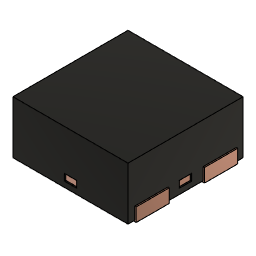
DPW0005A v3 (Autodesk Fusion 360 design; units mm, degrees)
Autodesk Fusion 360 part; units mm, degrees
sketch "Sketch1" plane through (0, 0, 0) normal (0, 0, 1) x (1, 0, 0)
  line L0 (0, 0) -> (0.85, 0)
  line L1 (0.85, 0) -> (0.85, 0.85)
  line L2 (0.85, 0.85) -> (0, 0.85)
  line L3 (0, 0.85) -> (0, 0)
  dimension "d1" = 0.85
  dimension "d2" = 0.85
  constraint horizontal L0
  constraint vertical L1
  constraint horizontal L2
  constraint vertical L3
  constraint coincident L0.start L3.end
  measures "d1" distance of L0.start L0.end
  measures "d2" distance of L0.start L2.end
extrude "Extrude1" add sketch "Sketch1" along normal blind 0.4
sketch "Sketch2" plane through (0, 0, 0) normal (0, 0, -1) x (1, 0, 0)
  line L0 (0, 0) -> (0, -0.85)
  line L1 (0, -0.85) -> (0.85, -0.85)
  line L2 (0.85, -0.85) -> (0.85, 0)
  line L3 (0.85, 0) -> (0, 0)
  line L4 (0.425, -0.85) -> (0.85, -0.85)
  line L5 (0.425, -0.85) -> (0.425, 0)
  line L6 (0.425, -0.425) -> (0.85, -0.425)
  line L7 (0.425, -0.425) -> (0, -0.425)
  line L8 (0.425, -0.425) -> (0.425, -0.241)
  line L9 (0.425, -0.425) -> (0.425, -0.609)
  line L10 (0.425, -0.425) -> (0.609, -0.425)
  line L11 (0.425, -0.425) -> (0.241, -0.425)
  line L12 (0.241, -0.425) -> (0.425, -0.241)
  line L13 (0.425, -0.241) -> (0.609, -0.425)
  line L14 (0.609, -0.425) -> (0.425, -0.609)
  line L15 (0.425, -0.609) -> (0.241, -0.425)
  line L16 (0, -0.425) -> (0, -0.555)
  line L17 (0, -0.425) -> (0, -0.295)
  line L18 (0.85, -0.425) -> (0.85, -0.295)
  line L19 (0.85, -0.425) -> (0.85, -0.555)
  line L20 (0.425, -0.85) -> (0.425, -0.75)
  line L21 (0.85, -0.425) -> (0.75, -0.425)
  line L22 (0.425, -0.75) -> (0.75, -0.425)
  line L23 (0.425, 0) -> (0.425, -0.1)
  line L24 (0.425, -0.1) -> (0.75, -0.425)
  line L25 (0, -0.425) -> (0.1, -0.425)
  line L26 (0.1, -0.425) -> (0.425, -0.1)
  line L27 (0.1, -0.425) -> (0.425, -0.75)
  line L28 (0, -0.555) -> (0.85, -0.555)
  line L29 (0.85, -0.295) -> (0, -0.295)
  line L30 (0, -0.85) -> (0, -0.8)
  line L31 (0, -0.8) -> (0.85, -0.8)
  line L32 (0.85, 0) -> (0.85, -0.05)
  line L33 (0, -0.05) -> (0.85, -0.05)
  line L34 (0.85, -0.05) -> (0, -0.05)
  line L35 (0.85, -0.8) -> (0.562, -0.8)
  line L36 (0, -0.8) -> (0.288, -0.8)
  line L37 (0, -0.05) -> (0.288, -0.05)
  line L38 (0.85, -0.05) -> (0.562, -0.05)
  line L39 (0.562, -0.8) -> (0.85, -0.512)
  line L40 (0.562, -0.8) -> (0.9693, -0.8) construction
  line L41 (0.288, -0.8) -> (0, -0.512)
  line L42 (0.562, -0.05) -> (0.85, -0.338)
  line L43 (0.288, -0.05) -> (0, -0.338)
  line L44 (0, -0.8) -> (0.239, -0.8)
  line L45 (0.239, -0.8) -> (0.239, -0.751)
  dimension "d7" = 0.184
  dimension "d8" = 0.184
  dimension "d9" = 0.184
  dimension "d10" = 0.184
  dimension "d11" = 0.13
  dimension "d12" = 0.13
  dimension "d13" = 0.13
  dimension "d14" = 0.13
  dimension "d15" = 0.288
  dimension "d16" = 0.288
  dimension "d17" = 0.288
  dimension "d18" = 0.288
  dimension "d19" = 45
  dimension "d20" = 90
  dimension "d21" = 90
  dimension "d22" = 0.239
  constraint midpoint L1 L4.start
  constraint coincident L1.end L2.start
  constraint perpendicular L4 L5
  constraint midpoint L5 L6.start
  constraint midpoint L2 L6.end
  constraint midpoint L0 L7.end
  constraint perpendicular L0 L7
  constraint perpendicular L7 L8
  constraint coincident L5 L9.end
  constraint perpendicular L5 L10
  constraint perpendicular L9 L11
  constraint perpendicular L7 L16
  constraint perpendicular L7 L17
  constraint perpendicular L6 L18
  constraint perpendicular L6 L19
  constraint coincident L5 L20.end
  constraint coincident L6 L21.end
  constraint coincident L5 L23.end
  constraint coincident L7 L25.end
  constraint coincident L0.end L1.start
  constraint coincident L0 L30.end
  constraint coincident L2 L31.end
  constraint perpendicular L2 L31
  constraint coincident L2.end L3.start
  constraint coincident L2 L32.end
  constraint perpendicular L3 L32
  constraint coincident L0 L33.start
  constraint perpendicular L2 L33
  constraint perpendicular L2 L35
  constraint perpendicular L30 L36
  constraint perpendicular L0 L37
  constraint perpendicular L32 L38
  constraint horizontal L40
  constraint coincident L19 L39.end
  constraint coincident L16 L41.end
  constraint coincident L18 L42.end
  constraint coincident L36 L44.end
  constraint coincident L41 L45.end
  constraint perpendicular L44 L45
  measures "d7" distance of L6.start L8.end
  measures "d8" distance of L6.start L9.end
  measures "d9" distance of L6.start L10.end
  measures "d10" distance of L6.start L11.end
  measures "d11" distance of L7.end L16.end
  measures "d12" distance of L7.end L17.end
  measures "d13" distance of L6.end L18.end
  measures "d14" distance of L6.end L19.end
  measures "d15" distance of L31.end L35.end
  measures "d16" distance of L30.end L36.end
  measures "d17" distance of L33.start L37.end
  measures "d18" distance of L32.end L38.end
  measures "d19" angle of L39 L40
  measures "d20" angle of L39 L41
  measures "d21" angle of L42 L43
  measures "d22" distance of L30.end L44.end
extrude "Extrude2" cut sketch "Sketch2" against normal blind 0.01 contours L0 L3 L5 L23 L33 L34 L37 | L2 L3 L5 L23 L32 L33 L34 L38 | L0 L17 L29 L43 | L5 L23 L26 L29 L33 L34 L43 | L5 L23 L24 L29 L33 L34 L42 | L0 L7 L17 L25 L26 L29 L43 | L5 L13 L24 L29 | L5 L12 L26 L29 | L0 L7 L16 L25 L27 L28 L41 | L7 L12 L26 L29 | L2 L18 L29 L42 | L2 L6 L18 L21 L24 L29 L42 | L6 L13 L24 L29 | L0 L16 L28 L41 | L7 L15 L27 L28 | L6 L14 L22 L28 | L2 L6 L19 L21 L22 L28 L39 | L5 L20 L27 L28 L31 L41 | L5 L15 L27 L28 | L5 L20 L22 L28 L31 L39 | L5 L14 L22 L28 | L0 L1 L5 L20 L30 L31 L36 L44 | L31 L36 L41 L45 | L2 L19 L28 L39 | L1 L2 L4 L5 L20 L31 L35
sketch "Sketch3" plane through (0, 0, 0) normal (-1, 0, 0) x (0, -1, 0)
  line L0 (-0.05, 0.01) -> (0, 0.01)
  line L1 (0, 0.01) -> (0, 0.4)
  line L2 (0, 0.4) -> (-0.85, 0.4)
  line L3 (-0.85, 0.4) -> (-0.85, 0.01)
  line L4 (-0.85, 0.01) -> (-0.8, 0.01)
  line L5 (-0.8, 0.01) -> (-0.8, 0)
  line L6 (-0.8, 0) -> (-0.555, 0)
  line L7 (-0.555, 0) -> (-0.555, 0.01)
  line L8 (-0.555, 0.01) -> (-0.295, 0.01)
  line L9 (-0.295, 0.01) -> (-0.295, 0)
  line L10 (-0.295, 0) -> (-0.05, 0)
  line L11 (-0.05, 0) -> (-0.05, 0.01)
  line L12 (-0.8, 0.01) -> (-0.8, 0.1)
  line L13 (-0.555, 0.01) -> (-0.555, 0.1)
  line L14 (-0.555, 0.1) -> (-0.8, 0.1)
  line L15 (-0.295, 0.01) -> (-0.295, 0.1)
  line L16 (-0.295, 0.1) -> (-0.05, 0.1)
  line L17 (-0.05, 0.1) -> (-0.05, 0.01)
  line L18 (-0.555, 0.1) -> (-0.47, 0.1)
  line L19 (-0.295, 0.1) -> (-0.38, 0.1)
  line L20 (-0.38, 0.1) -> (-0.47, 0.1)
  line L21 (-0.47, 0.1) -> (-0.47, 0.05)
  line L22 (-0.47, 0.05) -> (-0.38, 0.05)
  line L23 (-0.38, 0.05) -> (-0.38, 0.1)
  line L24 (-0.05, 0.1) -> (0, 0.1)
  line L25 (-0.8, 0.1) -> (-0.85, 0.1)
  dimension "d25" = 0.09
  constraint coincident L4.end L5.start
  constraint perpendicular L4 L12
  constraint coincident L7.end L8.start
  constraint perpendicular L8 L13
  constraint perpendicular L13 L14
  constraint coincident L8.end L9.start
  constraint perpendicular L8 L15
  constraint perpendicular L15 L16
  constraint coincident L0.start L11.end
  constraint perpendicular L15 L18
  constraint perpendicular L15 L19
  constraint perpendicular L15 L20
  constraint perpendicular L8 L21
  constraint perpendicular L21 L22
  constraint perpendicular L8 L23
  constraint coincident L1 L24.end
  constraint perpendicular L1 L24
  constraint coincident L3 L25.end
  constraint perpendicular L3 L25
  measures "d25" distance of L4.end L12.end
sketch "Sketch4" plane through (0, 0.85, 0) normal (0, 1, 0) x (-1, 0, 0)
  line L0 (-0.85, 0.01) -> (0, 0.01)
  line L1 (0, 0.01) -> (0, 0.4)
  line L2 (0, 0.4) -> (-0.85, 0.4)
  line L3 (-0.85, 0.4) -> (-0.85, 0.01)
  line L4 (0, 0.1) -> (-0.85, 0.1)
  line L5 (-0.425, 0.1) -> (-0.38, 0.1)
  line L6 (-0.425, 0.1) -> (-0.47, 0.1)
  line L7 (-0.47, 0.1) -> (-0.47, 0.05)
  line L8 (-0.47, 0.05) -> (-0.38, 0.05)
  line L9 (-0.38, 0.05) -> (-0.38, 0.1)
  constraint coincident L1 L4.start
  constraint coincident L3 L4.end
  constraint perpendicular L3 L4
  constraint midpoint L4 L5.start
  constraint coincident L4 L5.end
  constraint perpendicular L3 L5
  constraint coincident L4 L6.end
  constraint perpendicular L3 L6
  constraint perpendicular L5 L7
  constraint perpendicular L7 L8
  constraint perpendicular L8 L9
sketch "Sketch5" plane through (0, 0, 0) normal (0, -1, 0) x (1, 0, 0)
  line L0 (0, 0.01) -> (0.85, 0.01)
  line L1 (0.85, 0.01) -> (0.85, 0.4)
  line L2 (0.85, 0.4) -> (0, 0.4)
  line L3 (0, 0.4) -> (0, 0.01)
  line L4 (0, 0.1) -> (0.85, 0.1)
  line L5 (0.425, 0.1) -> (0.47, 0.1)
  line L6 (0.47, 0.1) -> (0.47, 0.05)
  line L7 (0.47, 0.05) -> (0.38, 0.05)
  line L8 (0.38, 0.05) -> (0.38, 0.1)
  constraint coincident L3 L4.start
  constraint coincident L1 L4.end
  constraint perpendicular L1 L4
  constraint midpoint L4 L5.start
  constraint coincident L4 L5.end
  constraint parallel L4 L5
  constraint perpendicular L4 L6
  constraint perpendicular L6 L7
  constraint coincident L4 L8.end
  constraint perpendicular L4 L8
sketch "Sketch6" plane through (0.85, 0, 0) normal (1, 0, 0) x (0, 1, 0)
  line L0 (0, 0.01) -> (0.05, 0.01)
  line L1 (0.05, 0.01) -> (0.05, 0)
  line L2 (0.05, 0) -> (0.295, 0)
  line L3 (0.295, 0) -> (0.295, 0.01)
  line L4 (0.295, 0.01) -> (0.555, 0.01)
  line L5 (0.555, 0.01) -> (0.555, 0)
  line L6 (0.555, 0) -> (0.8, 0)
  line L7 (0.8, 0) -> (0.8, 0.01)
  line L8 (0.8, 0.01) -> (0.85, 0.01)
  line L9 (0.85, 0.01) -> (0.85, 0.4)
  line L10 (0.85, 0.4) -> (0, 0.4)
  line L11 (0, 0.4) -> (0, 0.01)
  line L12 (0, 0.1) -> (0.85, 0.1)
  line L13 (0.425, 0.1) -> (0.47, 0.1)
  line L14 (0.47, 0.1) -> (0.47, 0.05)
  line L15 (0.47, 0.05) -> (0.38, 0.05)
  line L16 (0.38, 0.05) -> (0.38, 0.1)
  line L17 (0.555, 0.01) -> (0.555, 0.1)
  line L18 (0.8, 0.01) -> (0.8, 0.1)
  line L19 (0.295, 0.01) -> (0.295, 0.1)
  line L20 (0.05, 0.01) -> (0.05, 0.1)
  constraint coincident L11 L12.start
  constraint coincident L9 L12.end
  constraint perpendicular L9 L12
  constraint midpoint L12 L13.start
  constraint coincident L12 L13.end
  constraint perpendicular L9 L13
  constraint perpendicular L13 L14
  constraint perpendicular L9 L15
  constraint coincident L12 L16.end
  constraint perpendicular L12 L16
  constraint coincident L4.end L5.start
  constraint perpendicular L4 L17
  constraint coincident L7.end L8.start
  constraint perpendicular L8 L18
  constraint coincident L3.end L4.start
  constraint coincident L12 L19.end
  constraint perpendicular L12 L19
  constraint coincident L0.end L1.start
  constraint coincident L12 L20.end
  constraint perpendicular L12 L20
extrude "Extrude3" add sketch "Sketch4" along normal blind 0.01 contours L4 L5 L6 L7 L8 L9
extrude "Extrude4" add sketch "Sketch6" along normal blind 0.01 contours L1 L2 L3 L12 L19 L20 | L12 L13 L14 L15 L16 | L5 L6 L7 L12 L17 L18
extrude "Extrude5" add sketch "Sketch3" along normal blind 0.01 contours L9 L10 L11 L15 L16 L17 | L20 L21 L22 L23 | L5 L6 L7 L12 L13 L14
extrude "Extrude6" add sketch "Sketch5" along normal blind 0.01 contours L4 L5 L6 L7 L8
extrude "Extrude7" cut 1 faces at (0.86, 0.41, 0.0833) along direction (-1, 0, 0) blind 0.02
extrude "Extrude8" cut 1 faces at (0.41, -0.01, 0.0833) along direction (0, 1, 0) blind 0.02
extrude "Extrude9" cut 1 faces at (0.44, 0.86, 0.0833) along direction (0, -1, 0) blind 0.02
extrude "Extrude10" cut 1 faces at (-0.01, 0.44, 0.0833) along direction (1, 0, 0) blind 0.02
